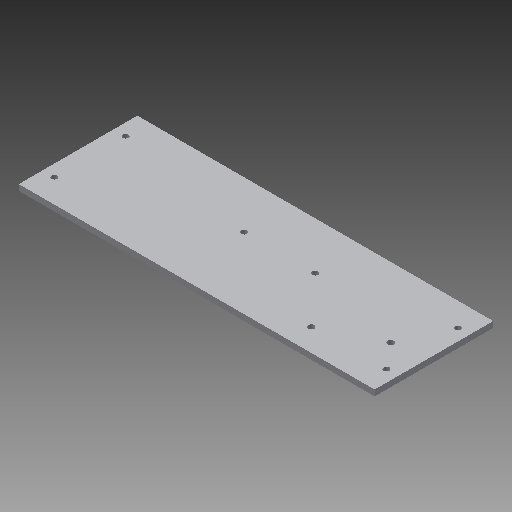
# Autodesk Inventor part: Power Mount Plate
Saved by Autodesk Inventor 2017 SP1 (Build 210196100, 196)
## iProperties
Created: 2016-04-02
Part Number: Power Mount Plate
Material: Aluminum 6061
Document SubType Name: Modeling
Designer: hwasserb
Density: 2.71 g/cm^3
Appearance: Aluminum - Flat
Author: hwasserb
Autodesk Inventor part; units mm, degrees
ref_plane "YZ Plane" through (0, 0, 0) normal (1, 0, 0) x (0, 1, 0)
ref_plane "XZ Plane" through (0, 0, 0) normal (0, 1, 0) x (-1, 0, 0)
ref_plane "XY Plane" through (0, 0, 0) normal (0, 0, 1) x (1, 0, 0)
sketch "Sketch1" plane through (0, 0, 0) normal (0, 1, 0) x (-1, 0, 0)
  line L0 (0, 0) -> (381, 0)
  line L1 (381, 0) -> (381, -127)
  line L2 (381, -127) -> (0, -127)
  line L3 (0, -127) -> (0, 0)
  dimension "d0" = 381
  dimension "d1" = 127
  constraints: 8 end point, 2 parallel, 1 horizontal, 1 perpendicular
  measures "d0" distance of L0.start L0.end
  measures "d1" distance of L2.end L0.start
extrude "Extrusion1" add sketch "Sketch1" along normal blind 6.35
sketch "Sketch2" plane through (0, 6.35, 0) normal (0, 1, 0) x (1, 0, 0)
  line L0 (0, 0) -> (0, 127) projected
  line L1 (0, 127) -> (-381, 127) projected
  line L2 (-381, 127) -> (-381, 0) projected
  point P0 (-368.3, 101.6)
  point P1 (-368.3, 25.4)
  point P2 (-12.7, 101.6)
  point P3 (-12.7, 25.4)
  dimension "d4" = 12.7
  dimension "d5" = 12.7
  dimension "d6" = 76.2
  dimension "d7" = 25.4
  constraints: 2 horizontal alignment, 2 vertical alignment
  measures "d4" distance from line of L2 point (-368.3, 101.6)
  measures "d5" distance from line of L0 point (-12.7, 101.6)
  measures "d6" distance of point (-12.7, 25.4) point (-12.7, 101.6)
  measures "d7" distance from line of L1 point (-368.3, 101.6)
hole "Hole1" at (-368.3, 6.35, -101.6) at (-368.3, 6.35, -25.4) at (-12.7, 6.35, -101.6) at (-12.7, 6.35, -25.4) direction (0, -1, 0) diameter 6.35 end through all
sketch "Sketch3" plane through (0, 6.35, 0) normal (0, 1, 0) x (1, 0, 0)
  line L0 (0, 127) -> (-381, 127) projected
  line L1 (-381, 127) -> (-381, 0) projected
  point P0 (-215.9, 76.2)
  point P1 (-139.7, 76.2)
  dimension "d15" = 76.2
  dimension "d16" = 50.8
  dimension "d17" = 165.1
  constraints: 1 horizontal alignment
  measures "d15" distance of point (-139.7, 76.2) point (-215.9, 76.2)
  measures "d16" distance from line of L0 point (-215.9, 76.2)
  measures "d17" distance from line of L1 point (-215.9, 76.2)
hole "Hole2" at (-215.9, 6.35, -76.2) at (-139.7, 6.35, -76.2) direction (0, -1, 0) diameter 6.5278 end through all
sketch "Sketch4" plane through (0, 6.35, 0) normal (0, 1, 0) x (1, 0, 0)
  line L0 (-381, 0) -> (0, 0) projected
  line L1 (0, 0) -> (0, 127) projected
  point P0 (-92.075, 24.13)
  point P1 (-34.925, 52.07)
  dimension "d25" = 57.15
  dimension "d26" = 27.94
  dimension "d27" = 24.13
  dimension "d28" = 34.925
  measures "d25" horizontal distance of point (-34.925, 52.07) point (-92.075, 24.13)
  measures "d26" vertical distance of point (-34.925, 52.07) point (-92.075, 24.13)
  measures "d27" distance from line of L0 point (-92.075, 24.13)
  measures "d28" distance from line of L1 point (-34.925, 52.07)
hole "Hole3" at (-92.075, 6.35, -24.13) at (-34.925, 6.35, -52.07) direction (0, -1, 0) diameter 6.858 end through all
body "Solid1"
